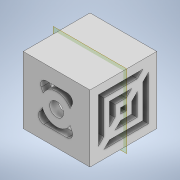
# Autodesk Inventor part: top-idler
Saved by Autodesk Inventor 2020.4 (Build 244396000, 396)
## iProperties
Created: 2021-04-07
Part Number: top-idler
Material: Generic
Document SubType Name: Modeling
Designer: AOB
Mass: 6.5435 g
Surface Area: 60.5468 cm^2
Volume: 6.5435 cm^3
Density: 1 g/cm^3
Appearance: Default
Author: AOB
Autodesk Inventor part; units mm, degrees
ref_plane "YZ Plane" through (0, 0, 0) normal (1, 0, 0) x (0, 1, 0)
ref_plane "XZ Plane" through (0, 0, 0) normal (0, 1, 0) x (-1, 0, 0)
ref_plane "XY Plane" through (0, 0, 0) normal (0, 0, 1) x (1, 0, 0)
sketch "Sketch1" plane through (0, 0, 0) normal (0, 0, 1) x (1, 0, 0)
  line L0 (0, 0) -> (18, 0) construction
  line L1 (18, 0) -> (18, -18) construction
  line L2 (18, -18) -> (0, -18) construction
  line L3 (0, -18) -> (0, 0) construction
  line L4 (-3, 3) -> (21, 3)
  line L5 (21, 3) -> (21, -21)
  line L6 (21, -21) -> (-3, -21)
  line L7 (-3, -21) -> (-3, 3)
  dimension "d0" = 18
  dimension "d1" = 18
  dimension "d2" = 24
  dimension "d3" = 24
  dimension "d4" = 3
  dimension "d5" = 3
  constraints: 16 end point, 4 parallel, 2 horizontal, 2 perpendicular
  measures "d0" distance of L0.start L0.end
  measures "d1" distance of L0.end L1.end
  measures "d2" distance of L5.end L6.end
  measures "d3" distance of L4.end L5.end
  measures "d4" distance between parallel lines of L4 L0
  measures "d5" distance between parallel lines of L7 L3
extrude "Extrusion1" add sketch "Sketch1" along normal blind 24
shell "Shell1" thickness 3 removed faces 0
sketch "Sketch3" plane through (0, 0, 24) normal (0, 0, 1) x (1, 0, 0)
  line L0 (21, 3) -> (-3, 3) projected
  line L1 (-3, 3) -> (-3, -21) projected
  line L2 (21, 3) -> (-3, -21)
  line L3 (-3, -21) -> (21, -21) projected
  line L4 (9, -9) -> (21, -21)
  line L5 (0, -18) -> (18, -18) construction
  line L6 (9, -18) -> (9, -16) construction
  line L7 (9, 0) -> (9, -2) construction
  line L8 (16, -2) -> (9, -16)
  line L9 (9, -16) -> (2, -2)
  line L10 (2, -2) -> (16, -2)
  line L11 (9, -2) -> (1, -16)
  line L12 (1, -16) -> (16, -16)
  line L13 (9, -2) -> (16, -16)
  point P0 (0, 0)
  point P1 (12.5, -9)
  point P2 (5.2667, -8.5333)
  dimension "d16" = 2
  dimension "d17" = 2
  constraints: 20 end point, 2 midpoint, 2 parallel, 2 point on line, 2 vertical
  measures "d16" distance of L6.start L6.end
  measures "d17" distance of L7.start L7.end
extrude "Extrusion3" cut sketch "Sketch3" against normal blind 10 contours L8 L13 L2 | L2 L13 L10 | L13 L8 L4 L2 | L2 L9 L11 L13 | L13 L4 L8 | L11 L9 L10 | L12 L11 L9 L2 | L2 L9 L12 | L4 L8 L9 L2 | L4 L12 L8
fillet "Fillet2" radius 2 4 edges at (2, -2, 22.5) (16, -2, 22.5) (16, -16, 22.5) (1, -16, 22.5)
sketch "Sketch6" plane through (0, 0, 24) normal (0, 0, 1) x (1, 0, 0)
  circle A0 centre (9, -9) radius 5.5
  circle A1 centre (9, -9) radius 2.5
  point P0 (0, 0)
  dimension "d26" = 11
  dimension "d27" = 5
  constraints: 2 centre point, 1 coincident
  measures "d26" diameter of A0
  measures "d27" diameter of A1
extrude "Extrusion5" add sketch "Sketch6" against normal blind 3
ref_plane "Work Plane1" through (0, 0, 12) normal (0, 0, -1) x (-1, 0, 0)
mirror "Mirror1" about plane through (0, 0, 12) normal (0, 0, -1) of "Extrusion5", "Fillet2", "Extrusion3"
sketch "Sketch7" plane through (-3, -21, 0) normal (-1, 0, 0) x (0, 0, 1)
  line L0 (5, 19) -> (19, 19)
  line L1 (19, 19) -> (19, 5)
  line L2 (19, 5) -> (5, 5)
  line L3 (5, 5) -> (5, 19)
  line L4 (0, 24) -> (24, 24) projected
  line L5 (0, 24) -> (0, 0) projected
  line L6 (2, 24) -> (0, 22)
  line L7 (0, 22) -> (22, 0)
  line L8 (0, 0) -> (24, 0) projected
  line L9 (24, 0) -> (24, 24) projected
  line L10 (24, 2) -> (2, 24)
  line L11 (3, 21) -> (21, 21) projected
  line L12 (3, 21) -> (3, 3) projected
  line L13 (21, 21) -> (21, 3) projected
  line L14 (3, 3) -> (21, 3) projected
  line L15 (7, 17) -> (17, 17)
  line L16 (17, 17) -> (17, 7)
  line L17 (17, 7) -> (7, 7)
  line L18 (7, 7) -> (7, 17)
  line L19 (9, 15) -> (15, 15)
  line L20 (15, 15) -> (15, 9)
  line L21 (15, 9) -> (9, 9)
  line L22 (9, 9) -> (9, 15)
  line L23 (11, 13) -> (13, 13)
  line L24 (13, 13) -> (13, 11)
  line L25 (13, 11) -> (11, 11)
  line L26 (11, 11) -> (11, 13)
  point P0 (15, 11)
  point P1 (17, 9)
  point P2 (9, 17)
  point P3 (11, 15)
  point P4 (9, 13)
  point P5 (7, 15)
  point P6 (15, 7)
  point P7 (13, 9)
  point P8 (19, 3)
  point P9 (17, 5)
  point P10 (5, 17)
  point P11 (3, 19)
  point P12 (21, 5)
  point P13 (5, 21)
  point P14 (7, 19)
  point P15 (19, 7)
  dimension "d30" = 14
  dimension "d31" = 14
  dimension "d33" = 2
  dimension "d34" = 2
  constraints: 38 end point, 9 parallel, 4 horizontal, 4 perpendicular, 4 point on line
  measures "d30" distance of L1.end L2.end
  measures "d31" distance of L0.end L1.end
  measures "d33" distance between parallel lines of L14 L2
  measures "d34" distance between parallel lines of L1 L13
extrude "Extrusion6" cut sketch "Sketch7" against normal through all contours L10 L11 L13 L1 L0 | L3 L2 L7 L14 L12 | L15 L16 L10 L20 L19 | L7 L22 L21 L17 L18 | L24 L25 L26 L23
body "Solid1"
